Autodesk Inventor part; units mm, degrees
(part 3 of 3)
  arc A728 (-43.5459, 16.289) -> (-42.8903, 15.993) centre (-41.0276, 20.9926) ccw
  arc A729 (-44.0216, 17.9437) -> (-43.4305, 17.4605) centre (-40.8808, 21.1827) ccw
  arc A730 (-44.7219, 17.1379) -> (-44.1577, 16.6713) centre (-40.8999, 21.1842) ccw
  arc A731 (-44.1577, 16.6713) -> (-43.5459, 16.289) centre (-40.9969, 21.0499) ccw
  arc A732 (-43.4305, 17.4605) -> (-42.777, 17.0941) centre (-41.064, 20.9154) ccw
  arc A733 (-41.2579, 16.7048) -> (-41.0583, 16.6972) centre (-41.095, 18.3595) ccw
  arc A734 (-42.0544, 16.8434) -> (-41.2579, 16.7048) centre (-40.7232, 22.1353) ccw
  arc A735 (-42.8903, 15.993) -> (-41.2076, 15.6459) centre (-40.9253, 21.2672) ccw
  arc A736 (-42.777, 17.0941) -> (-42.0544, 16.8434) centre (-40.9868, 21.0875) ccw
  arc A737 (-41.2232, 18.4187) -> (-40.8534, 18.4163) centre (-41.0092, 22.9779) ccw
  arc A738 (-42.4468, 18.85) -> (-41.9954, 18.6104) centre (-40.9017, 21.2163) ccw
  arc A739 (-41.9954, 18.6104) -> (-41.5087, 18.4563) centre (-40.9069, 21.2039) ccw
  arc A740 (-41.5087, 18.4563) -> (-41.2232, 18.4187) centre (-41.1431, 20.1255) ccw
  line L106 (-47.3871, 15.9419) -> (-47.2208, 15.752)
  line L107 (-48.0091, 15.3693) -> (-47.3871, 15.9419)
  arc A741 (-47.2208, 15.752) -> (-46.2453, 14.8022) centre (-40.787, 21.3841) ccw
  arc A742 (-46.2453, 14.8022) -> (-45.131, 14.0188) centre (-40.777, 21.3962) ccw
  arc A743 (-45.5736, 15.6227) -> (-45.3081, 15.4041) centre (-43.271, 18.1489) ccw
  arc A744 (-45.977, 16.0001) -> (-45.5736, 15.6227) centre (-31.4221, 31.1485) ccw
  line L108 (-46.5959, 16.6722) -> (-45.9786, 17.2551)
  line L109 (-46.5311, 16.5791) -> (-46.5959, 16.6722)
  arc A745 (-46.5311, 16.5791) -> (-46.3689, 16.385) centre (-45.3427, 17.4073) ccw
  arc A746 (-46.3689, 16.385) -> (-45.977, 16.0001) centre (-28.5706, 34.1163) ccw
  arc A747 (-39.2532, 13.0523) -> (-37.9823, 13.4278) centre (-40.8354, 20.7457) ccw
  arc A748 (-40.0911, 12.9248) -> (-39.2532, 13.0523) centre (-40.9016, 21.0679) ccw
  arc A749 (-40.9902, 13.9498) -> (-40.5238, 13.9555) centre (-40.9642, 30.9285) ccw
  arc A750 (-40.5238, 13.9555) -> (-40.2018, 13.9767) centre (-40.629, 18.009) ccw
  arc A751 (-40.2018, 13.9767) -> (-39.6005, 14.0671) centre (-40.9339, 20.8877) ccw
  arc A752 (-41.2076, 15.6459) -> (-39.5165, 15.8286) centre (-40.9361, 21.0509) ccw
  arc A753 (-41.0583, 16.6972) -> (-40.7499, 16.7094) centre (-41.2542, 25.5623) ccw
  arc A754 (-38.9986, 14.211) -> (-38.4115, 14.404) centre (-41.0253, 21.3635) ccw
  arc A755 (-39.6005, 14.0671) -> (-38.9986, 14.211) centre (-41.0306, 21.382) ccw
  arc A756 (-44.4844, 14.8686) -> (-43.6198, 14.4534) centre (-40.9436, 21.1344) ccw
  arc A757 (-45.3081, 15.4041) -> (-44.4844, 14.8686) centre (-40.5869, 21.7656) ccw
  arc A758 (-43.6198, 14.4534) -> (-42.7099, 14.1578) centre (-40.957, 21.1008) ccw
  arc A759 (-45.131, 14.0188) -> (-43.9174, 13.4283) centre (-40.8575, 21.2597) ccw
  arc A760 (-44.8003, 11.951) -> (-43.313, 11.4624) centre (-40.9786, 21.0755) ccw
  arc A761 (-46.1906, 12.6676) -> (-44.8003, 11.951) centre (-40.9858, 21.0582) ccw
  arc A762 (-43.9174, 13.4283) -> (-42.6466, 13.0523) centre (-41.0712, 20.7129) ccw
  arc A763 (-43.313, 11.4624) -> (-41.7507, 11.2077) centre (-40.8736, 21.5081) ccw
  line L110 (-48.6312, 14.7966) -> (-48.0091, 15.3693)
  line L111 (-48.5373, 14.6782) -> (-48.6312, 14.7966)
  arc A764 (-48.5373, 14.6782) -> (-48.3495, 14.4607) centre (-45.8896, 16.7752) ccw
  arc A765 (-48.3495, 14.4607) -> (-48.057, 14.1585) centre (-37.5805, 24.5936) ccw
  arc A766 (-48.057, 14.1585) -> (-47.7404, 13.8498) centre (-37.3233, 24.8498) ccw
  arc A767 (-47.7404, 13.8498) -> (-47.4641, 13.6007) centre (-42.494, 19.3899) ccw
  arc A768 (-47.4641, 13.6007) -> (-46.1906, 12.6676) centre (-40.7886, 21.3762) ccw
  arc A769 (-38.5756, 17.3904) -> (-38.1676, 17.6912) centre (-41.641, 21.9759) ccw
  arc A770 (-38.9731, 17.1587) -> (-38.5756, 17.3904) centre (-40.6602, 20.5087) ccw
  arc A771 (-39.2289, 17.0457) -> (-38.9731, 17.1587) centre (-40.2179, 19.6304) ccw
  arc A772 (-39.5165, 15.8286) -> (-37.9591, 16.5288) centre (-40.9482, 21.0955) ccw
  arc A773 (-39.5614, 16.9281) -> (-39.2289, 17.0457) centre (-41.6999, 23.5038) ccw
  arc A774 (-39.9011, 16.8271) -> (-39.5614, 16.9281) centre (-41.7094, 23.5332) ccw
  arc A775 (-40.1799, 16.7662) -> (-39.9011, 16.8271) centre (-40.6703, 19.6799) ccw
  arc A776 (-40.4304, 16.7335) -> (-40.1799, 16.7662) centre (-40.7514, 20.1611) ccw
  arc A777 (-39.3522, 18.9228) -> (-38.983, 19.2368) centre (-41.1244, 21.3807) ccw
  arc A778 (-40.7499, 16.7094) -> (-40.4304, 16.7335) centre (-41.2496, 25.483) ccw
  arc A779 (-37.285, 11.8775) -> (-35.9421, 12.5287) centre (-40.9194, 21.0828) ccw
  arc A780 (-37.294, 14.9384) -> (-36.7902, 15.2627) centre (-40.5426, 20.5375) ccw
  arc A781 (-36.772, 14.0162) -> (-35.6594, 14.7986) centre (-41.1077, 21.3631) ccw
  arc A782 (-37.8545, 14.6418) -> (-37.294, 14.9384) centre (-41.3698, 21.9632) ccw
  arc A783 (-35.9421, 12.5287) -> (-34.6975, 13.3804) centre (-41.1319, 21.4479) ccw
  arc A784 (-38.4115, 14.404) -> (-37.8545, 14.6418) centre (-40.8225, 20.8234) ccw
  arc A785 (-37.9823, 13.4278) -> (-36.772, 14.0162) centre (-41.0146, 21.2053) ccw
  arc A786 (-36.7902, 15.2627) -> (-36.3178, 15.6328) centre (-40.5561, 20.5565) ccw
  arc A787 (-36.3178, 15.6328) -> (-35.8513, 16.0668) centre (-41.6997, 21.8851) ccw
  arc A788 (-35.8513, 16.0668) -> (-35.6869, 16.2341) centre (-49.5707, 29.7156) ccw
  arc A789 (-35.6869, 16.2341) -> (-35.5379, 16.39) centre (-45.6213, 25.8806) ccw
  arc A790 (-37.79, 18.0273) -> (-37.4844, 18.3655) centre (-40.3313, 20.6309) ccw
  arc A791 (-37.376, 18.5054) -> (-37.3338, 18.5623) centre (-47.3292, 25.9345) ccw
  arc A792 (-37.3338, 18.5623) -> (-37.3309, 18.5711) centre (-37.3457, 18.5711) ccw
  arc A793 (-37.3309, 18.5711) -> (-37.3402, 18.5926) centre (-37.3604, 18.5711) ccw
  arc A794 (-37.3402, 18.5926) -> (-37.9358, 19.1523) centre (-1609.827, -1654.0056) ccw
  arc A795 (-37.9358, 19.1523) -> (-38.5237, 19.7043) centre (-850.002, -845.2296) ccw
  arc A796 (-38.5237, 19.7043) -> (-38.5639, 19.7294) centre (-38.6075, 19.615) ccw
  arc A797 (-38.5639, 19.7294) -> (-38.5781, 19.7265) centre (-38.5687, 19.7168) ccw
  arc A798 (-38.5781, 19.7265) -> (-38.6109, 19.6926) centre (-38.075, 19.2071) ccw
  arc A799 (-35.5379, 16.39) -> (-35.4148, 16.5223) centre (-46.5034, 26.7109) ccw
  arc A800 (-35.4148, 16.5223) -> (-35.3698, 16.5784) centre (-35.8109, 16.8862) ccw
  line L112 (-35.3053, 16.6708) -> (-35.3698, 16.5784)
  line L113 (-35.9223, 17.2541) -> (-35.3053, 16.6708)
  arc A801 (-37.9591, 16.5288) -> (-36.6652, 17.6853) centre (-41.1435, 21.3939) ccw
  arc A802 (-37.4256, 18.4403) -> (-37.376, 18.5054) centre (-40.8459, 21.0954) ccw
  arc A803 (-41.7203, 19.6952) -> (-41.3041, 19.5023) centre (-40.9224, 20.8718) ccw
  arc A804 (-42.057, 20.0117) -> (-41.7203, 19.6952) centre (-40.8992, 20.9061) ccw
  arc A805 (-42.2759, 20.4145) -> (-42.057, 20.0117) centre (-40.9189, 20.8909) ccw
  arc A806 (-42.351, 20.8575) -> (-42.2759, 20.4145) centre (-41.0214, 20.8549) ccw
  arc A807 (-42.2073, 21.4686) -> (-42.351, 20.8575) centre (-40.9678, 20.8548) ccw
  arc A808 (-40.6171, 22.2151) -> (-41.2375, 22.2276) centre (-40.9535, 20.9235) ccw
  arc A809 (-40.2585, 22.0718) -> (-40.6171, 22.2151) centre (-41.0066, 20.7196) ccw
  arc A810 (-39.5827, 20.565) -> (-39.5945, 21.1925) centre (-40.8932, 20.8542) ccw
  arc A811 (-39.9614, 21.8481) -> (-40.2585, 22.0718) centre (-40.9034, 20.9061) ccw
  arc A812 (-39.7377, 21.5511) -> (-39.9614, 21.8481) centre (-40.9034, 20.9061) ccw
  arc A813 (-39.5945, 21.1925) -> (-39.7377, 21.5511) centre (-41.0899, 20.8029) ccw
  arc A814 (-41.2375, 22.2276) -> (-41.8076, 21.9596) centre (-40.937, 20.8476) ccw
  arc A815 (-41.8076, 21.9596) -> (-42.2073, 21.4686) centre (-40.9266, 20.8344) ccw
  line L114 (-31.75, 0) -> (-31.75, 87.9)
  line L115 (-28.9873, 15.9412) -> (-29.6096, 15.3693)
  line L116 (-29.6096, 15.3693) -> (-30.2319, 14.7974)
  line L117 (-30.2319, 14.7974) -> (-30.1343, 14.6715)
  line L118 (-28.8207, 15.7516) -> (-28.9873, 15.9412)
  arc A816 (-30.1343, 14.6715) -> (-29.9306, 14.439) centre (-28.0795, 16.2658) ccw
  arc A817 (-29.9306, 14.439) -> (-29.5272, 14.0392) centre (-11.6488, 32.4803) ccw
  arc A818 (-28.8207, 15.7516) -> (-27.8406, 14.7986) centre (-22.2817, 21.4964) ccw
  arc A819 (-28.8025, 13.3804) -> (-27.5579, 12.5287) centre (-22.3681, 21.4479) ccw
  arc A820 (-29.1063, 13.6411) -> (-28.8025, 13.3804) centre (-25.3293, 17.7351) ccw
  arc A821 (-29.5272, 14.0392) -> (-29.1063, 13.6411) centre (-13.2395, 30.8395) ccw
  arc A822 (-23.2925, 11.2049) -> (-22.9286, 11.1845) centre (-22.6866, 18.7517) ccw
  arc A823 (-22.5184, 11.1783) -> (-22.1093, 11.186) centre (-22.5404, 23.2644) ccw
  arc A824 (-24.788, 11.4351) -> (-23.2925, 11.2049) centre (-22.4575, 21.6039) ccw
  arc A825 (-22.9286, 11.1845) -> (-22.5184, 11.1783) centre (-22.5405, 23.318) ccw
  arc A826 (-27.8406, 14.7986) -> (-26.728, 14.0162) centre (-22.3923, 21.3631) ccw
  arc A827 (-27.1822, 15.6328) -> (-26.7098, 15.2627) centre (-22.9439, 20.5565) ccw
  arc A828 (-26.7098, 15.2627) -> (-26.206, 14.9384) centre (-22.9574, 20.5375) ccw
  arc A829 (-26.206, 14.9384) -> (-25.6455, 14.6418) centre (-22.1302, 21.9632) ccw
  arc A830 (-27.5579, 12.5287) -> (-26.215, 11.8775) centre (-22.5806, 21.0828) ccw
  arc A831 (-26.728, 14.0162) -> (-25.5177, 13.4278) centre (-22.4854, 21.2053) ccw
  arc A832 (-25.6455, 14.6418) -> (-25.0885, 14.404) centre (-22.6775, 20.8234) ccw
  arc A833 (-26.215, 11.8775) -> (-24.788, 11.4351) centre (-22.572, 21.1045) ccw
  arc A834 (-23.4089, 12.9248) -> (-22.5501, 12.8822) centre (-22.5501, 21.5531) ccw
  arc A835 (-22.9762, 13.9555) -> (-22.5098, 13.9498) centre (-22.5358, 30.9285) ccw
  arc A836 (-24.2468, 13.0523) -> (-23.4089, 12.9248) centre (-22.5984, 21.0679) ccw
  arc A837 (-23.2982, 13.9767) -> (-22.9762, 13.9555) centre (-22.871, 18.009) ccw
  arc A838 (-25.5177, 13.4278) -> (-24.2468, 13.0523) centre (-22.6646, 20.7457) ccw
  arc A839 (-24.5014, 14.211) -> (-23.8995, 14.0671) centre (-22.4694, 21.382) ccw
  arc A840 (-25.0885, 14.404) -> (-24.5014, 14.211) centre (-22.4747, 21.3635) ccw
  arc A841 (-23.8995, 14.0671) -> (-23.2982, 13.9767) centre (-22.5661, 20.8877) ccw
  line L119 (-26.8348, 17.6853) -> (-26.9607, 17.8373)
  line L120 (-26.9607, 17.8373) -> (-27.5777, 17.2541)
  arc A842 (-27.6487, 16.0668) -> (-27.1822, 15.6328) centre (-21.8003, 21.8851) ccw
  arc A843 (-27.8131, 16.2341) -> (-27.6487, 16.0668) centre (-13.9293, 29.7156) ccw
  arc A844 (-27.9621, 16.39) -> (-27.8131, 16.2341) centre (-17.8787, 25.8806) ccw
  arc A845 (-28.0852, 16.5223) -> (-27.9621, 16.39) centre (-16.9966, 26.7109) ccw
  arc A846 (-28.1302, 16.5784) -> (-28.0852, 16.5223) centre (-27.6891, 16.8862) ccw
  line L121 (-28.1947, 16.6708) -> (-28.1302, 16.5784)
  arc A847 (-26.8348, 17.6853) -> (-25.5409, 16.5288) centre (-22.3565, 21.3939) ccw
  line L122 (-27.5777, 17.2541) -> (-28.1947, 16.6708)
  arc A848 (-25.71, 18.0273) -> (-25.3324, 17.6912) centre (-21.8751, 21.9562) ccw
  arc A849 (-26.0744, 18.4403) -> (-26.0156, 18.3655) centre (-19.8293, 23.2881) ccw
  arc A850 (-26.0156, 18.3655) -> (-25.71, 18.0273) centre (-23.1687, 20.6309) ccw
  arc A851 (-26.124, 18.5054) -> (-26.0744, 18.4403) centre (-22.6541, 21.0954) ccw
  arc A852 (-26.1691, 18.5711) -> (-26.1662, 18.5623) centre (-26.1543, 18.5711) ccw
  arc A853 (-26.1598, 18.5926) -> (-26.1691, 18.5711) centre (-26.1396, 18.5711) ccw
  arc A854 (-26.1662, 18.5623) -> (-26.124, 18.5054) centre (-16.1708, 25.9345) ccw
  arc A855 (-23.9835, 15.8286) -> (-22.2924, 15.6459) centre (-22.5639, 21.0509) ccw
  arc A856 (-22.7501, 16.7094) -> (-22.4417, 16.6972) centre (-22.2458, 25.5623) ccw
  arc A857 (-23.0696, 16.7335) -> (-22.7501, 16.7094) centre (-22.2504, 25.483) ccw
  arc A858 (-23.3201, 16.7662) -> (-23.0696, 16.7335) centre (-22.7486, 20.1611) ccw
  arc A859 (-23.5989, 16.8271) -> (-23.3201, 16.7662) centre (-22.8297, 19.6799) ccw
  arc A860 (-23.9386, 16.9281) -> (-23.5989, 16.8271) centre (-21.7906, 23.5332) ccw
  arc A861 (-24.2711, 17.0457) -> (-23.9386, 16.9281) centre (-21.8001, 23.5038) ccw
  arc A862 (-24.5269, 17.1587) -> (-24.2711, 17.0457) centre (-23.2821, 19.6304) ccw
  arc A863 (-24.9244, 17.3904) -> (-24.5269, 17.1587) centre (-22.8398, 20.5087) ccw
  arc A864 (-25.3324, 17.6912) -> (-24.9244, 17.3904) centre (-21.859, 21.9759) ccw
  arc A865 (-25.5409, 16.5288) -> (-23.9835, 15.8286) centre (-22.5518, 21.0955) ccw
  arc A866 (-24.8106, 19.5908) -> (-24.517, 19.2368) centre (-22.7785, 20.9773) ccw
  arc A867 (-24.8106, 19.5908) -> (-24.8511, 19.6468) centre (-25.8767, 18.8634) ccw
  arc A868 (-24.8511, 19.6468) -> (-24.8891, 19.6926) centre (-25.4156, 19.2156) ccw
  arc A869 (-24.517, 19.2368) -> (-24.1478, 18.9228) centre (-22.3756, 21.3807) ccw
  arc A870 (-25.5642, 19.1523) -> (-26.1598, 18.5926) centre (1546.327, -1654.0056) ccw
  arc A871 (-24.9763, 19.7043) -> (-25.5642, 19.1523) centre (786.502, -845.2296) ccw
  arc A872 (-24.9361, 19.7294) -> (-24.9763, 19.7043) centre (-24.8925, 19.615) ccw
  arc A873 (-24.9219, 19.7265) -> (-24.9361, 19.7294) centre (-24.9313, 19.7168) ccw
  arc A874 (-24.8891, 19.6926) -> (-24.9219, 19.7265) centre (-25.425, 19.2071) ccw
  arc A875 (-23.0157, 18.4439) -> (-22.6466, 18.4163) centre (-22.4907, 22.9814) ccw
  arc A876 (-23.2992, 18.501) -> (-23.0157, 18.4439) centre (-22.8166, 20.1643) ccw
  arc A877 (-24.1478, 18.9228) -> (-23.7319, 18.6707) centre (-22.3638, 21.3971) ccw
  arc A878 (-23.7319, 18.6707) -> (-23.2992, 18.501) centre (-22.5894, 20.9474) ccw
  arc A879 (-20.723, 17.0941) -> (-20.0695, 17.4605) centre (-22.436, 20.9154) ccw
  arc A880 (-21.4456, 16.8434) -> (-20.723, 17.0941) centre (-22.5132, 21.0875) ccw
  arc A881 (-20.6097, 15.993) -> (-19.9541, 16.289) centre (-22.4724, 20.9926) ccw
  arc A882 (-22.2421, 16.7048) -> (-21.4456, 16.8434) centre (-22.7768, 22.1353) ccw
  arc A883 (-22.4417, 16.6972) -> (-22.2421, 16.7048) centre (-22.405, 18.3595) ccw
  arc A884 (-21.6912, 12.9248) -> (-20.8534, 13.0523) centre (-22.5018, 21.0679) ccw
  arc A885 (-20.8534, 13.0523) -> (-19.5826, 13.4283) centre (-22.4288, 20.7129) ccw
  arc A886 (-22.5501, 12.8822) -> (-21.6912, 12.9248) centre (-22.5501, 21.5531) ccw
  arc A887 (-19.5826, 13.4283) -> (-18.369, 14.0188) centre (-22.6425, 21.2597) ccw
  arc A888 (-19.8802, 14.4534) -> (-19.0156, 14.8686) centre (-22.5564, 21.1344) ccw
  arc A889 (-19.0156, 14.8686) -> (-18.1919, 15.4041) centre (-22.9131, 21.7656) ccw
  arc A890 (-20.7901, 14.1578) -> (-19.8802, 14.4534) centre (-22.543, 21.1008) ccw
  arc A891 (-21.7493, 13.9791) -> (-20.7901, 14.1578) centre (-22.6851, 21.664) ccw
  arc A892 (-22.0476, 13.9567) -> (-21.7493, 13.9791) centre (-22.1391, 17.1799) ccw
  arc A893 (-22.5098, 13.9498) -> (-22.0476, 13.9567) centre (-22.5361, 31.1776) ccw
  arc A894 (-22.2924, 15.6459) -> (-20.6097, 15.993) centre (-22.5747, 21.2672) ccw
  arc A895 (-23.1428, 19.5961) -> (-22.5205, 19.461) centre (-22.5413, 20.8649) ccw
  arc A896 (-23.6436, 19.9925) -> (-23.1428, 19.5961) centre (-22.5342, 20.88) ccw
  arc A897 (-23.9173, 20.565) -> (-23.6436, 19.9925) centre (-22.551, 20.8665) ccw
  arc A898 (-22.2622, 19.4873) -> (-22.1959, 19.5023) centre (-22.3824, 20.1718) ccw
  arc A899 (-22.3484, 19.4743) -> (-22.2622, 19.4873) centre (-22.5824, 21.3102) ccw
  arc A900 (-22.4392, 19.4648) -> (-22.3484, 19.4743) centre (-22.596, 21.4166) ccw
  arc A901 (-22.5205, 19.461) -> (-22.4392, 19.4648) centre (-22.5389, 20.7066) ccw
  arc A902 (-21.7797, 19.6952) -> (-21.443, 20.0117) centre (-22.6008, 20.9061) ccw
  arc A903 (-21.5046, 18.6104) -> (-21.0532, 18.85) centre (-22.5983, 21.2163) ccw
  arc A904 (-22.1959, 19.5023) -> (-21.7797, 19.6952) centre (-22.5776, 20.8718) ccw
  arc A905 (-21.9913, 18.4563) -> (-21.5046, 18.6104) centre (-22.5931, 21.2039) ccw
  arc A906 (-22.2768, 18.4187) -> (-21.9913, 18.4563) centre (-22.3569, 20.1255) ccw
  arc A907 (-22.6466, 18.4163) -> (-22.2768, 18.4187) centre (-22.4908, 22.9779) ccw
  arc A908 (-19.4784, 17.9437) -> (-19.2886, 18.1354) centre (-24.0751, 22.6842) ccw
  arc A909 (-20.0695, 17.4605) -> (-19.4784, 17.9437) centre (-22.6192, 21.1827) ccw
  arc A910 (-19.3423, 16.6713) -> (-18.7781, 17.1379) centre (-22.6001, 21.1842) ccw
  arc A911 (-19.9541, 16.289) -> (-19.3423, 16.6713) centre (-22.5031, 21.0499) ccw
  arc A912 (-18.6997, 11.951) -> (-17.3094, 12.6676) centre (-22.5142, 21.0582) ccw
  arc A913 (-18.369, 14.0188) -> (-17.2547, 14.8022) centre (-22.723, 21.3962) ccw
  arc A914 (-17.3094, 12.6676) -> (-16.0359, 13.6007) centre (-22.7114, 21.3762) ccw
  arc A915 (-17.2547, 14.8022) -> (-16.2792, 15.752) centre (-22.713, 21.3841) ccw
  arc A916 (-19.535, 19.1514) -> (-20.1215, 19.703) centre (-773.3736, -781.7675) ccw
  arc A917 (-20.6547, 19.1654) -> (-20.3253, 19.5443) centre (-22.4898, 21.0935) ccw
  arc A918 (-21.0532, 18.85) -> (-20.6547, 19.1654) centre (-22.5801, 21.1884) ccw
  arc A919 (-19.2886, 18.1354) -> (-19.1076, 18.3339) centre (-23.9951, 22.6081) ccw
  arc A920 (-19.1076, 18.3339) -> (-18.9499, 18.5179) centre (-28.4315, 26.4879) ccw
  arc A921 (-18.9499, 18.5179) -> (-18.9311, 18.5696) centre (-19.0114, 18.5696) ccw
  arc A922 (-18.9311, 18.5696) -> (-18.9407, 18.5918) centre (-18.9617, 18.5696) ccw
  arc A923 (-18.9407, 18.5918) -> (-19.535, 19.1514) centre (-1491.7979, -1545.0609) ccw
  arc A924 (-20.2704, 19.6179) -> (-20.3253, 19.5443) centre (-18.3798, 18.1517) ccw
  arc A925 (-20.2204, 19.6785) -> (-20.2704, 19.6179) centre (-19.2538, 18.8295) ccw
  arc A926 (-20.1215, 19.703) -> (-20.163, 19.7291) centre (-20.2086, 19.6103) ccw
  arc A927 (-20.163, 19.7291) -> (-20.1773, 19.7258) centre (-20.1677, 19.7168) ccw
  arc A928 (-20.1773, 19.7258) -> (-20.2204, 19.6785) centre (-18.9101, 18.5276) ccw
  arc A929 (-21.443, 20.0117) -> (-21.2241, 20.4145) centre (-22.5811, 20.8909) ccw
  arc A930 (-21.2241, 20.4145) -> (-21.149, 20.8575) centre (-22.4786, 20.8549) ccw
  arc A931 (-18.7781, 17.1379) -> (-18.265, 17.6856) centre (-22.997, 21.6045) ccw
  line L123 (-18.1388, 17.838) -> (-18.265, 17.6856)
  line L124 (-17.5214, 17.2551) -> (-18.1388, 17.838)
  arc A932 (-18.1919, 15.4041) -> (-17.9264, 15.6227) centre (-20.229, 18.1489) ccw
  arc A933 (-17.9264, 15.6227) -> (-17.523, 16.0001) centre (-32.0779, 31.1485) ccw
  line L125 (-16.9041, 16.6722) -> (-17.5214, 17.2551)
  arc A934 (-17.523, 16.0001) -> (-17.1311, 16.385) centre (-34.9294, 34.1163) ccw
  arc A935 (-17.1311, 16.385) -> (-16.9689, 16.5791) centre (-18.1573, 17.4073) ccw
  line L126 (-16.9689, 16.5791) -> (-16.9041, 16.6722)
  line L127 (-16.1129, 15.9419) -> (-16.2792, 15.752)
  line L128 (-15.4909, 15.3693) -> (-16.1129, 15.9419)
  arc A936 (-16.0359, 13.6007) -> (-15.7596, 13.8498) centre (-21.006, 19.3899) ccw
  arc A937 (-15.7596, 13.8498) -> (-15.443, 14.1585) centre (-26.1767, 24.8498) ccw
  arc A938 (-15.443, 14.1585) -> (-15.1505, 14.4607) centre (-25.9195, 24.5936) ccw
  arc A939 (-15.1505, 14.4607) -> (-14.9627, 14.6782) centre (-17.6104, 16.7752) ccw
  line L129 (-14.9627, 14.6782) -> (-14.8688, 14.7966)
  line L130 (-14.8688, 14.7966) -> (-15.4909, 15.3693)
  arc A940 (-22.1093, 11.186) -> (-21.7493, 11.2077) centre (-22.3704, 18.5023) ccw
  arc A941 (-21.7493, 11.2077) -> (-20.187, 11.4624) centre (-22.6264, 21.5081) ccw
  arc A942 (-20.187, 11.4624) -> (-18.6997, 11.951) centre (-22.5214, 21.0755) ccw
  arc A943 (-22.2625, 22.2276) -> (-22.8829, 22.2151) centre (-22.5465, 20.9235) ccw
  arc A944 (-22.8829, 22.2151) -> (-23.2415, 22.0718) centre (-22.4934, 20.7196) ccw
  arc A945 (-23.2415, 22.0718) -> (-23.5386, 21.8481) centre (-22.5966, 20.9061) ccw
  arc A946 (-23.5386, 21.8481) -> (-23.7623, 21.5511) centre (-22.5966, 20.9061) ccw
  arc A947 (-23.7623, 21.5511) -> (-23.9055, 21.1925) centre (-22.4101, 20.8029) ccw
  arc A948 (-23.9055, 21.1925) -> (-23.9173, 20.565) centre (-22.6068, 20.8542) ccw
  arc A949 (-21.149, 20.8575) -> (-21.2927, 21.4686) centre (-22.5322, 20.8548) ccw
  arc A950 (-21.6924, 21.9596) -> (-22.2625, 22.2276) centre (-22.563, 20.8476) ccw
  arc A951 (-21.2927, 21.4686) -> (-21.6924, 21.9596) centre (-22.5734, 20.8344) ccw
  line L131 (-50.2817, 78.9621) -> (-51.492, 78.9621)
  line L132 (-51.492, 78.9621) -> (-51.492, 75.4711)
  line L133 (-51.492, 75.4711) -> (-52.8011, 75.4711)
  line L134 (-52.8011, 75.4711) -> (-52.8011, 78.9621)
  line L135 (-52.8011, 78.9621) -> (-57.2883, 78.9621)
  line L136 (-57.2883, 78.9621) -> (-57.2883, 80.3947)
  line L137 (-57.2883, 80.3947) -> (-52.7435, 85.6311)
  line L138 (-52.7435, 85.6311) -> (-51.492, 85.6311)
  line L139 (-51.492, 85.6311) -> (-51.492, 80.0571)
  line L140 (-51.492, 80.0571) -> (-50.2817, 80.0571)
  line L141 (-50.2817, 80.0571) -> (-50.2817, 78.9621)
  line L142 (-52.8011, 80.0571) -> (-52.8011, 84.0256)
  line L143 (-52.8011, 84.0256) -> (-56.218, 80.0571)
  line L144 (-56.218, 80.0571) -> (-52.8011, 80.0571)
  line L145 (-13.2183, 10.2825) -> (-12.008, 10.2825)
  line L146 (-12.008, 10.2825) -> (-12.008, 13.7735)
  line L147 (-12.008, 13.7735) -> (-10.6989, 13.7735)
  line L148 (-10.6989, 13.7735) -> (-10.6989, 10.2825)
  line L149 (-10.6989, 10.2825) -> (-6.2117, 10.2825)
  line L150 (-6.2117, 10.2825) -> (-6.2117, 8.8499)
  line L151 (-6.2117, 8.8499) -> (-10.7565, 3.6135)
  line L152 (-10.7565, 3.6135) -> (-12.008, 3.6135)
  line L153 (-12.008, 3.6135) -> (-12.008, 9.1875)
  line L154 (-12.008, 9.1875) -> (-13.2183, 9.1875)
  line L155 (-13.2183, 9.1875) -> (-13.2183, 10.2825)
  line L156 (-10.6989, 9.1875) -> (-10.6989, 5.219)
  line L157 (-10.6989, 5.219) -> (-7.282, 9.1875)
  line L158 (-7.282, 9.1875) -> (-10.6989, 9.1875)
  line L159 (-50.2817, 78.9621) -> (-51.492, 78.9621)
  line L160 (-51.492, 78.9621) -> (-51.492, 75.4711)
  line L161 (-51.492, 75.4711) -> (-52.8011, 75.4711)
  line L162 (-52.8011, 75.4711) -> (-52.8011, 78.9621)
  line L163 (-52.8011, 78.9621) -> (-57.2883, 78.9621)
  line L164 (-57.2883, 78.9621) -> (-57.2883, 80.3947)
  line L165 (-57.2883, 80.3947) -> (-52.7435, 85.6311)
  line L166 (-52.7435, 85.6311) -> (-51.492, 85.6311)
  line L167 (-51.492, 85.6311) -> (-51.492, 80.0571)
  line L168 (-51.492, 80.0571) -> (-50.2817, 80.0571)
  line L169 (-50.2817, 80.0571) -> (-50.2817, 78.9621)
  line L170 (-52.8011, 80.0571) -> (-52.8011, 84.0256)
  line L171 (-52.8011, 84.0256) -> (-56.218, 80.0571)
  line L172 (-56.218, 80.0571) -> (-52.8011, 80.0571)
  line L173 (-13.2183, 10.2825) -> (-12.008, 10.2825)
  line L174 (-12.008, 10.2825) -> (-12.008, 13.7735)
  line L175 (-12.008, 13.7735) -> (-10.6989, 13.7735)
  line L176 (-10.6989, 13.7735) -> (-10.6989, 10.2825)
  line L177 (-10.6989, 10.2825) -> (-6.2117, 10.2825)
  line L178 (-6.2117, 10.2825) -> (-6.2117, 8.8499)
  line L179 (-6.2117, 8.8499) -> (-10.7565, 3.6135)
  line L180 (-10.7565, 3.6135) -> (-12.008, 3.6135)
  line L181 (-12.008, 3.6135) -> (-12.008, 9.1875)
  line L182 (-12.008, 9.1875) -> (-13.2183, 9.1875)
  line L183 (-13.2183, 9.1875) -> (-13.2183, 10.2825)
  line L184 (-10.6989, 9.1875) -> (-10.6989, 5.219)
  line L185 (-10.6989, 5.219) -> (-7.282, 9.1875)
  line L186 (-7.282, 9.1875) -> (-10.6989, 9.1875)
  point P0 (-40.9176, 72.907)
  point P1 (-30.7426, 155.7595)
  point P2 (-40.9176, 72.907)
  point P3 (-53.7479, 68.8958)
  point P4 (-53.7479, 68.8958)
  point P5 (-9.7521, 20.0042)
  point P6 (-9.7521, 20.0042)
  point P7 (-34.6793, 73.1484)
  point P8 (-33.3657, 74.2285)
  point P9 (-33.5694, 74.461)
  point P10 (-33.9729, 74.8609)
  point P11 (-34.3937, 75.2589)
  point P12 (-34.6975, 75.5196)
  point P13 (-35.9423, 76.3714)
  point P14 (-37.2838, 77.022)
  point P15 (-38.712, 77.465)
  point P16 (-40.2075, 77.6951)
  point P17 (-40.5713, 77.7155)
  point P18 (-40.982, 77.7217)
  point P19 (-41.3906, 77.714)
  point P20 (-41.7508, 77.6923)
  point P21 (-43.3127, 77.4377)
  point P22 (-44.7921, 76.9524)
  point P23 (-46.1906, 76.2324)
  point P24 (-47.4641, 75.2993)
  point P25 (-47.7404, 75.0502)
  point P26 (-48.0565, 74.7419)
  point P27 (-48.3495, 74.4393)
  point P28 (-48.5373, 74.2218)
  point P29 (-47.2208, 73.148)
  point P30 (-46.2474, 74.0961)
  point P31 (-45.1309, 74.8813)
  point P32 (-43.9176, 75.4716)
  point P33 (-42.6463, 75.8477)
  point P34 (-41.8086, 75.9752)
  point P35 (-40.9499, 76.0178)
  point P36 (-40.0912, 75.9752)
  point P37 (-39.2534, 75.8477)
  point P38 (-37.9822, 75.4721)
  point P39 (-36.7719, 74.8838)
  point P40 (-35.6595, 74.1015)
  point P41 (-36.6652, 71.2147)
  point P42 (-35.3698, 72.3216)
  point P43 (-35.4148, 72.3777)
  point P44 (-35.5378, 72.5099)
  point P45 (-35.6869, 72.6659)
  point P46 (-35.8513, 72.8332)
  point P47 (-36.3178, 73.2672)
  point P48 (-36.7913, 73.638)
  point P49 (-37.294, 73.9616)
  point P50 (-37.8545, 74.2582)
  point P51 (-38.4116, 74.496)
  point P52 (-38.9975, 74.6887)
  point P53 (-39.6006, 74.8329)
  point P54 (-40.2018, 74.9233)
  point P55 (-40.5238, 74.9445)
  point P56 (-40.9893, 74.9502)
  point P57 (-41.4524, 74.9433)
  point P58 (-41.7507, 74.9209)
  point P59 (-42.7098, 74.7422)
  point P60 (-43.6211, 74.446)
  point P61 (-44.4844, 74.0314)
  point P62 (-45.3081, 73.4959)
  point P63 (-45.5736, 73.2773)
  point P64 (-45.977, 72.8999)
  point P65 (-46.3689, 72.515)
  point P66 (-46.5311, 72.3209)
  point P67 (-45.235, 71.2144)
  point P68 (-44.7219, 71.7621)
  point P69 (-44.1577, 72.2288)
  point P70 (-43.5454, 72.6112)
  point P71 (-42.8905, 72.9069)
  point P72 (-41.2075, 73.2541)
  point P73 (-39.5166, 73.0714)
  point P74 (-37.9591, 72.3712)
  point P75 (-38.6489, 69.2532)
  point P76 (-38.6109, 69.2075)
  point P77 (-38.5781, 69.1735)
  point P78 (-38.5639, 69.1706)
  point P79 (-38.5237, 69.1957)
  point P80 (-37.9363, 69.7472)
  point P81 (-37.3402, 70.3074)
  point P82 (-37.3309, 70.3289)
  point P83 (-37.3338, 70.3377)
  point P84 (-37.376, 70.3946)
  point P85 (-37.4255, 70.4597)
  point P86 (-37.4844, 70.5345)
  point P87 (-37.79, 70.8727)
  point P88 (-38.1661, 71.2076)
  point P89 (-38.5757, 71.5096)
  point P90 (-38.9731, 71.7413)
  point P91 (-39.2289, 71.8543)
  point P92 (-39.5619, 71.9721)
  point P93 (-39.9011, 72.0729)
  point P94 (-40.1799, 72.1338)
  point P95 (-40.4304, 72.1665)
  point P96 (-40.7485, 72.1905)
  point P97 (-41.0583, 72.2028)
  point P98 (-41.2579, 72.1952)
  point P99 (-42.0544, 72.0566)
  point P100 (-42.777, 71.8059)
  point P101 (-43.4306, 71.4394)
  point P102 (-44.0216, 70.9563)
  point P103 (-44.2111, 70.7649)
  point P104 (-44.3924, 70.5661)
  point P105 (-44.5501, 70.3821)
  point P106 (-44.5689, 70.3304)
  point P107 (-44.5593, 70.3082)
  point P108 (-43.9647, 69.7483)
  point P109 (-43.3785, 69.197)
  point P110 (-43.337, 69.1709)
  point P111 (-43.3227, 69.1742)
  point P112 (-43.2796, 69.2215)
  point P113 (-43.2296, 69.2821)
  point P114 (-43.1747, 69.3557)
  point P115 (-42.8453, 69.7346)
  point P116 (-42.4468, 70.0501)
  point P117 (-41.9953, 70.2897)
  point P118 (-41.5087, 70.4437)
  point P119 (-41.2232, 70.4813)
  point P120 (-40.8534, 70.4837)
  point P121 (-40.4843, 70.4561)
  point P122 (-40.2008, 70.399)
  point P123 (-39.7681, 70.2293)
  point P124 (-39.3522, 69.9772)
  point P125 (-38.983, 69.6632)
  point P126 (-38.6894, 69.3092)
  point P127 (-41.2378, 69.4127)
  point P128 (-41.3041, 69.3977)
  point P129 (-41.7204, 69.2048)
  point P130 (-42.057, 68.8884)
  point P131 (-42.2759, 68.4855)
  point P132 (-42.351, 68.0425)
  point P133 (-42.2073, 67.4314)
  point P134 (-41.8076, 66.9404)
  point P135 (-41.2375, 66.6724)
  point P136 (-40.6171, 66.6849)
  point P137 (-40.2585, 66.8282)
  point P138 (-39.9614, 67.0519)
  point P139 (-39.7377, 67.3489)
  point P140 (-39.5945, 67.7075)
  point P141 (-39.5827, 68.335)
  point P142 (-39.8563, 68.9074)
  point P143 (-40.3573, 69.3039)
  point P144 (-40.9795, 69.439)
  point P145 (-41.0608, 69.4352)
  point P146 (-41.1516, 69.4257)
  point P147 (-10.5703, 22.8165)
  point P148 (-10.4026, 22.4657)
  point P149 (-10.0955, 22.2226)
  point P150 (-9.7141, 22.1398)
  point P151 (-9.6642, 22.1422)
  point P152 (-9.6086, 22.1479)
  point P153 (-9.5557, 22.1559)
  point P154 (-9.5151, 22.1652)
  point P155 (-9.2599, 22.2834)
  point P156 (-9.0536, 22.4773)
  point P157 (-8.9194, 22.7243)
  point P158 (-8.8734, 22.9959)
  point P159 (-8.9615, 23.3705)
  point P160 (-9.2064, 23.6715)
  point P161 (-9.5559, 23.8357)
  point P162 (-9.9363, 23.8281)
  point P163 (-10.1561, 23.7402)
  point P164 (-10.3382, 23.6031)
  point P165 (-10.4753, 23.421)
  point P166 (-10.5631, 23.2012)
  point P167 (-11.1179, 22.2194)
  point P168 (-11.1427, 22.2537)
  point P169 (-11.1661, 22.2818)
  point P170 (-11.1862, 22.3026)
  point P171 (-11.1949, 22.3043)
  point P172 (-11.2195, 22.289)
  point P173 (-11.5796, 21.9509)
  point P174 (-11.945, 21.6075)
  point P175 (-11.9503, 21.5909)
  point P176 (-11.923, 21.5541)
  point P177 (-11.8927, 21.5141)
  point P178 (-11.8566, 21.4683)
  point P179 (-11.6693, 21.2609)
  point P180 (-11.4387, 21.0557)
  point P181 (-11.1876, 20.8705)
  point P182 (-10.944, 20.7285)
  point P183 (-10.7872, 20.6592)
  point P184 (-10.5831, 20.587)
  point P185 (-10.3752, 20.5253)
  point P186 (-10.2042, 20.4879)
  point P187 (-10.0507, 20.4678)
  point P188 (-9.8557, 20.4531)
  point P189 (-9.6658, 20.4456)
  point P190 (-9.5434, 20.4503)
  point P191 (-9.0551, 20.5352)
  point P192 (-8.6122, 20.6889)
  point P193 (-8.2116, 20.9135)
  point P194 (-7.8493, 21.2097)
  point P195 (-7.7331, 21.327)
  point P196 (-7.622, 21.4489)
  point P197 (-7.5253, 21.5617)
  point P198 (-7.5138, 21.5934)
  point P199 (-7.5197, 21.607)
  dimension "d103" = 8.4153
  dimension "d105" = 0.508
  dimension "d106" = 0.508
  dimension "d107" = -2.9972
  dimension "d108" = 4.8735
  dimension "d111" = 2.9972
  dimension "d112" = -2.9972
  constraints: 1904 point on circle, 1329 symmetric about line, 952 centre point, 238 end point, 4 midpoint, 412 other
  measures "d103" distance of L12.end L14.start
  measures "d105" distance between parallel lines of L15 L7
  measures "d106" distance between parallel lines of L16 L11
  measures "d107" vertical distance of point (-30.743, 155.76) A129.centre
  measures "d108" vertical distance of point (-40.918, 72.907) A265.centre
  measures "d111" vertical distance of point (-53.748, 68.896) A401.centre
  measures "d112" vertical distance of point (-9.752, 20.004) A537.centre
extrude "Extrusion20" add sketch "Sketch17" along normal blind 0.4 contours A167 A166 A165 A164 A163 A162 A161 A160 A159 A158 A157 A156 L40 L39 L38 L37 A155 A154 A153 A152 A151 A150 A149 A148 A147 A146 A145 A144 L36 L35 L34 L33 A143 A142 A141 A140 A139 A138 A137 A136 | A199 A198 A197 A196 A195 A194 A193 A192 A191 A190 A189 A188 A187 A186 A185 A184 L48 L47 L46 L45 A183 A182 A181 A180 A179 A178 A177 A176 L44 L43 L42 L41 A175 A174 A173 A172 A171 A170 A169 A168 | A251 A250 A249 A248 A247 A246 A245 A244 A243 A242 A241 A240 A239 A238 A237 A236 A235 A234 A233 A232 A231 A230 A229 A228 A227 A226 A225 A224 A223 A222 A221 A220 A219 A218 A217 A216 A215 A214 A213 A212 A211 A210 A209 A208 A207 A206 A205 A204 A203 A202 A201 A200 | A271 A270 A269 A268 A267 A266 A265 A264 A263 A262 A261 A260 A259 A258 A257 A256 A255 A254 A253 A252 | A303 A302 A301 A300 A299 A298 A297 A296 A295 A294 A293 A292 L56 L55 L54 L53 A291 A290 A289 A288 A287 A286 A285 A284 A283 A282 A281 A280 L52 L51 L50 L49 A279 A278 A277 A276 A275 A274 A273 A272 | A335 A334 A333 A332 A331 A330 A329 A328 A327 A326 A325 A324 A323 A322 A321 A320 L64 L63 L62 L61 A319 A318 A317 A316 A315 A314 A313 A312 L60 L59 L58 L57 A311 A310 A309 A308 A307 A306 A305 A304 | A387 A386 A385 A384 A383 A382 A381 A380 A379 A378 A377 A376 A375 A374 A373 A372 A371 A370 A369 A368 A367 A366 A365 A364 A363 A362 A361 A360 A359 A358 A357 A356 A355 A354 A353 A352 A351 A350 A349 A348 A347 A346 A345 A344 A343 A342 A341 A340 A339 A338 A337 A336 | A407 A406 A405 A404 A403 A402 A401 A400 A399 A398 A397 A396 A395 A394 A393 A392 A391 A390 A389 A388 | A439 A438 A437 A436 A435 A434 A433 A432 A431 A430 A429 A428 L72 L71 L70 L69 A427 A426 A425 A424 A423 A422 A421 A420 A419 A418 A417 A416 L68 L67 L66 L65 A415 A414 A413 A412 A411 A410 A409 A408 | A471 A470 A469 A468 A467 A466 A465 A464 A463 A462 A461 A460 A459 A458 A457 A456 L80 L79 L78 L77 A455 A454 A453 A452 A451 A450 A449 A448 L76 L75 L74 L73 A447 A446 A445 A444 A443 A442 A441 A440 | A523 A522 A521 A520 A519 A518 A517 A516 A515 A514 A513 A512 A511 A510 A509 A508 A507 A506 A505 A504 A503 A502 A501 A500 A499 A498 A497 A496 A495 A494 A493 A492 A491 A490 A489 A488 A487 A486 A485 A484 A483 A482 A481 A480 A479 A478 A477 A476 A475 A474 A473 A472 | A543 A542 A541 A540 A539 A538 A537 A536 A535 A534 A533 A532 A531 A530 A529 A528 A527 A526 A525 A524 | L82 L83 L84 A544 A545 A547 A548 A647 A643 A560 A559 A558 A553 A549 A550 A627 A624 A625 A632 A631 A630 A629 A628 L95 L94 L91 L90 A605 A606 A623 A626 A551 A554 A557 A612 A611 A649 A645 A546 L85 | A622 A620 A621 A607 A608 A610 A609 L93 L92 L89 L88 A591 A594 A595 A592 A599 A616 A636 A665 L86 L87 L97 L96 A664 A663 A653 A652 A651 A650 A644 A646 A648 A618 A619 A615 A614 A613 A556 A555 A552 | A667 A668 A669 A670 A671 A679 A678 A672 A673 A675 A676 A677 A674 A567 A566 A565 A564 A563 A562 A561 | A568 A569 A570 A662 A661 A660 A659 A658 A657 A656 A655 A666 A590 A654 A589 A633 A634 A635 A637 A638 A639 A640 A642 A617 A597 A598 A600 A596 A593 A584 A585 A586 A587 A588 A571 A572 A579 A578 A577 A576 A575 A574 A573 A602 A603 A604 A601 A580 A581 A583 A582 A641 | L98 L99 L100 A680 A681 A683 A684 A783 A779 A696 A695 A694 A689 A685 A686 A763 A760 A761 A768 A767 A766 A765 A764 L111 L110 L107 L106 A741 A742 A759 A762 A687 A690 A693 A748 A747 A785 A781 A682 L101 | A758 A756 A757 A743 A744 A746 A745 L109 L108 L105 L104 A727 A730 A731 A728 A735 A752 A772 A801 L102 L103 L113 L112 A800 A799 A789 A788 A787 A786 A780 A782 A784 A754 A755 A751 A750 A749 A692 A691 A688 | A803 A804 A805 A806 A807 A815 A814 A808 A809 A811 A812 A813 A810 A703 A702 A701 A700 A699 A698 A697 | A704 A705 A706 A798 A797 A796 A795 A794 A793 A792 A791 A802 A726 A790 A725 A769 A770 A771 A773 A774 A775 A776 A778 A753 A733 A734 A736 A732 A729 A720 A721 A722 A723 A724 A707 A708 A715 A714 A713 A712 A711 A710 A709 A738 A739 A740 A737 A716 A717 A719 A718 A777 | L118 A818 A826 A831 A838 A836 A834 A886 A884 A885 A887 A913 A915 L127 L128 L130 L129 A939 A938 A937 A936 A914 A912 A942 A941 A940 A823 A825 A822 A824 A833 A830 A819 A820 A821 A817 A816 L117 L116 L115 | A842 A843 A844 A845 A846 L121 L122 L120 L119 A847 A865 A855 A894 A881 A911 A910 A931 L123 L124 L125 L126 A935 A934 A933 A932 A889 A888 A890 A891 A892 A893 A835 A837 A841 A839 A840 A832 A829 A828 A827 | A850 A849 A851 A854 A852 A853 A870 A871 A872 A873 A874 A868 A867 A866 A869 A877 A878 A876 A875 A907 A906 A905 A903 A918 A917 A924 A925 A928 A927 A926 A916 A923 A922 A921 A920 A919 A908 A909 A879 A880 A882 A883 A856 A857 A858 A859 A860 A861 A862 A863 A864 A848 | A896 A897 A948 A947 A946 A945 A944 A943 A950 A951 A949 A930 A929 A902 A904 A898 A899 A900 A901 A895 | L131 L132 L133 L134 L135 L136 L137 L138 L139 L140 L141 | L145 L146 L147 L148 L149 L150 L151 L152 L153 L154 L155 bodies 2
sketch "Sketch18" plane through (0, 0, -0.2) normal (0, 0, -1) x (-1, 0, 0)
  line L0 (0, 0) -> (-63.5, 0)
  line L1 (-63.5, 0) -> (-63.5, 88.9)
  line L2 (-63.5, 88.9) -> (0, 88.9)
  line L3 (0, 88.9) -> (0, 0)
  constraints: 8 end point, 2 parallel, 1 horizontal, 1 perpendicular
extrude "Extrusion21" add sketch "Sketch18" along normal blind 0.4 bodies 3
fillet "Fillet2" radius 3.175 8 edges at (63.5, 0, 0.2) (63.5, 88.9, 0.2) (0, 0, 0.2) (0, 88.9, 0.2) (63.5, 0, -0.3) (63.5, 88.9, -0.3) (0, 0, -0.3) (0, 88.9, -0.3)
extrude "Extrusion22" cut sketch "Sketch17" along normal blind 0.4 contours A167 A166 A165 A164 A163 A162 A161 A160 A159 A158 A157 A156 L40 L39 L38 L37 A155 A154 A153 A152 A151 A150 A149 A148 A147 A146 A145 A144 L36 L35 L34 L33 A143 A142 A141 A140 A139 A138 A137 A136 | A199 A198 A197 A196 A195 A194 A193 A192 A191 A190 A189 A188 A187 A186 A185 A184 L48 L47 L46 L45 A183 A182 A181 A180 A179 A178 A177 A176 L44 L43 L42 L41 A175 A174 A173 A172 A171 A170 A169 A168 | A251 A250 A249 A248 A247 A246 A245 A244 A243 A242 A241 A240 A239 A238 A237 A236 A235 A234 A233 A232 A231 A230 A229 A228 A227 A226 A225 A224 A223 A222 A221 A220 A219 A218 A217 A216 A215 A214 A213 A212 A211 A210 A209 A208 A207 A206 A205 A204 A203 A202 A201 A200 | A271 A270 A269 A268 A267 A266 A265 A264 A263 A262 A261 A260 A259 A258 A257 A256 A255 A254 A253 A252 | A303 A302 A301 A300 A299 A298 A297 A296 A295 A294 A293 A292 L56 L55 L54 L53 A291 A290 A289 A288 A287 A286 A285 A284 A283 A282 A281 A280 L52 L51 L50 L49 A279 A278 A277 A276 A275 A274 A273 A272 | A335 A334 A333 A332 A331 A330 A329 A328 A327 A326 A325 A324 A323 A322 A321 A320 L64 L63 L62 L61 A319 A318 A317 A316 A315 A314 A313 A312 L60 L59 L58 L57 A311 A310 A309 A308 A307 A306 A305 A304 | A387 A386 A385 A384 A383 A382 A381 A380 A379 A378 A377 A376 A375 A374 A373 A372 A371 A370 A369 A368 A367 A366 A365 A364 A363 A362 A361 A360 A359 A358 A357 A356 A355 A354 A353 A352 A351 A350 A349 A348 A347 A346 A345 A344 A343 A342 A341 A340 A339 A338 A337 A336 | A407 A406 A405 A404 A403 A402 A401 A400 A399 A398 A397 A396 A395 A394 A393 A392 A391 A390 A389 A388 | A439 A438 A437 A436 A435 A434 A433 A432 A431 A430 A429 A428 L72 L71 L70 L69 A427 A426 A425 A424 A423 A422 A421 A420 A419 A418 A417 A416 L68 L67 L66 L65 A415 A414 A413 A412 A411 A410 A409 A408 | A471 A470 A469 A468 A467 A466 A465 A464 A463 A462 A461 A460 A459 A458 A457 A456 L80 L79 L78 L77 A455 A454 A453 A452 A451 A450 A449 A448 L76 L75 L74 L73 A447 A446 A445 A444 A443 A442 A441 A440 | A523 A522 A521 A520 A519 A518 A517 A516 A515 A514 A513 A512 A511 A510 A509 A508 A507 A506 A505 A504 A503 A502 A501 A500 A499 A498 A497 A496 A495 A494 A493 A492 A491 A490 A489 A488 A487 A486 A485 A484 A483 A482 A481 A480 A479 A478 A477 A476 A475 A474 A473 A472 | A543 A542 A541 A540 A539 A538 A537 A536 A535 A534 A533 A532 A531 A530 A529 A528 A527 A526 A525 A524 | L82 L83 L84 A544 A545 A547 A548 A647 A643 A560 A559 A558 A553 A549 A550 A627 A624 A625 A632 A631 A630 A629 A628 L95 L94 L91 L90 A605 A606 A623 A626 A551 A554 A557 A612 A611 A649 A645 A546 L85 | A622 A620 A621 A607 A608 A610 A609 L93 L92 L89 L88 A591 A594 A595 A592 A599 A616 A636 A665 L86 L87 L97 L96 A664 A663 A653 A652 A651 A650 A644 A646 A648 A618 A619 A615 A614 A613 A556 A555 A552 | A667 A668 A669 A670 A671 A679 A678 A672 A673 A675 A676 A677 A674 A567 A566 A565 A564 A563 A562 A561 | A568 A569 A570 A662 A661 A660 A659 A658 A657 A656 A655 A666 A590 A654 A589 A633 A634 A635 A637 A638 A639 A640 A642 A617 A597 A598 A600 A596 A593 A584 A585 A586 A587 A588 A571 A572 A579 A578 A577 A576 A575 A574 A573 A602 A603 A604 A601 A580 A581 A583 A582 A641 | L98 L99 L100 A680 A681 A683 A684 A783 A779 A696 A695 A694 A689 A685 A686 A763 A760 A761 A768 A767 A766 A765 A764 L111 L110 L107 L106 A741 A742 A759 A762 A687 A690 A693 A748 A747 A785 A781 A682 L101 | A758 A756 A757 A743 A744 A746 A745 L109 L108 L105 L104 A727 A730 A731 A728 A735 A752 A772 A801 L102 L103 L113 L112 A800 A799 A789 A788 A787 A786 A780 A782 A784 A754 A755 A751 A750 A749 A692 A691 A688 | A803 A804 A805 A806 A807 A815 A814 A808 A809 A811 A812 A813 A810 A703 A702 A701 A700 A699 A698 A697 | A704 A705 A706 A798 A797 A796 A795 A794 A793 A792 A791 A802 A726 A790 A725 A769 A770 A771 A773 A774 A775 A776 A778 A753 A733 A734 A736 A732 A729 A720 A721 A722 A723 A724 A707 A708 A715 A714 A713 A712 A711 A710 A709 A738 A739 A740 A737 A716 A717 A719 A718 A777 | L118 A818 A826 A831 A838 A836 A834 A886 A884 A885 A887 A913 A915 L127 L128 L130 L129 A939 A938 A937 A936 A914 A912 A942 A941 A940 A823 A825 A822 A824 A833 A830 A819 A820 A821 A817 A816 L117 L116 L115 | A842 A843 A844 A845 A846 L121 L122 L120 L119 A847 A865 A855 A894 A881 A911 A910 A931 L123 L124 L125 L126 A935 A934 A933 A932 A889 A888 A890 A891 A892 A893 A835 A837 A841 A839 A840 A832 A829 A828 A827 | A850 A849 A851 A854 A852 A853 A870 A871 A872 A873 A874 A868 A867 A866 A869 A877 A878 A876 A875 A907 A906 A905 A903 A918 A917 A924 A925 A928 A927 A926 A916 A923 A922 A921 A920 A919 A908 A909 A879 A880 A882 A883 A856 A857 A858 A859 A860 A861 A862 A863 A864 A848 | A896 A897 A948 A947 A946 A945 A944 A943 A950 A951 A949 A930 A929 A902 A904 A898 A899 A900 A901 A895 | L131 L132 L133 L134 L135 L136 L137 L138 L139 L140 L141 | L145 L146 L147 L148 L149 L150 L151 L152 L153 L154 L155 bodies 3
